Probe Tip 2mm M1.6_v5 (Autodesk Fusion 360 design; units mm, degrees)
Autodesk Fusion 360 part; units mm, degrees
sketch "Sketch1" plane through (0, 0, 0) normal (0, 0, 1) x (1, 0, 0)
  line L0 (0, 0) -> (1, 0)
  line L1 (1, 0) -> (1, 6)
  line L2 (0.8, 19.3) -> (1, 6)
  line L3 (0, 0) -> (0, 20.9)
  circle A0 centre (0, 19.9) radius 1
  line L4 (0, 0) -> (0.8, 0)
  line L5 (0.8, 0) -> (0.8, -2)
  line L6 (0.8, -2) -> (0, -2)
  line L7 (0, -2) -> (0, 0)
  dimension "d1" = 1
  dimension "d2" = 6
  dimension "d3" = 0.8
  dimension "d4" = 20.9
  dimension "d5" = 2
  dimension "d6" = 0.8
  dimension "d7" = 2
  constraint coincident L0.start L3.start
  constraint horizontal L0
  constraint perpendicular L0 L1
  constraint perpendicular L0 L3
  constraint coincident L3.end A0
  constraint coincident L2.start A0
  constraint horizontal L4
  constraint vertical L5
  constraint horizontal L6
  constraint vertical L7
  measures "d1" distance of L0.start L0.end
  measures "d2" distance of L0.end L1.end
  measures "d3" horizontal distance of L0.start L2.start
  measures "d4" distance of L0.start L3.end
  measures "d5" diameter of A0
  measures "d6" distance of L0.start L4.end
  measures "d7" distance of L0.start L6.end
revolve "Revolve1" add sketch "Sketch1" angle 360 about axis through (0, 0, 0) along (0, 1, 0) contours L0 L1 L2 L3 A0 L4 makes body 1 in component "Shank"
revolve "Revolve1'" add sketch "Sketch1" angle 360 about axis through (0, -2, 0) along (0, 1, 0) separate body contours L0 L4 L5 L6 L7 makes body 2 in component "Thread"
revolve "Revolve1''" add sketch "Sketch1" angle 360 about axis through (0, 0, 0) along (0, 1, 0) separate body contours L3 A0 picked at (0.4113, 19.9934) makes body 3 in component "Ball"
thread "Thread1" "ISO Metric profile 1.6 M1.6x0.35 6g" major diameter 1.5385 minor diameter 1.1385 pitch 0.35 angle 60 resizes the face on face at (0.799, -0.6667, 0.0399) on bodies 2 in component "Thread"
component "Shank" placed x (1, 0, 0) y (0, 1, 0) z (0, 0, 1) at (0, 0, 0)
component "Thread" placed x (1, 0, 0) y (0, 1, 0) z (0, 0, 1) at (0, 0, 0)
component "Ball" placed x (1, 0, 0) y (0, 1, 0) z (0, 0, 1) at (0, 0, 0)
